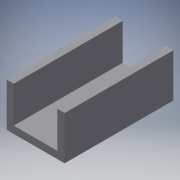
# Autodesk Inventor part: anclaje
Saved by Autodesk Inventor 2018 (Build 220112000, 112)
## iProperties
Created: 2021-07-06
Part Number: anclaje
Material: Genérico
Document SubType Name: Modeling
Designer: GABRIEL
Density: 1 g/cm^3
Appearance: Valor por defecto
Author: GABRIEL
Autodesk Inventor part; units mm, degrees
ref_plane "YZ Plane" through (0, 0, 0) normal (1, 0, 0) x (0, 1, 0)
ref_plane "XZ Plane" through (0, 0, 0) normal (0, 1, 0) x (-1, 0, 0)
ref_plane "XY Plane" through (0, 0, 0) normal (0, 0, 1) x (1, 0, 0)
sketch "Boceto1" plane through (0, 0, 0) normal (0, 1, 0) x (-1, 0, 0)
  line L0 (0, 0) -> (-80, 0)
  line L1 (-80, 0) -> (-80, -40)
  line L2 (-80, -40) -> (0, -40)
  line L3 (0, -40) -> (0, 0)
  line L4 (-10, 0) -> (-70, 0)
  line L5 (-70, 0) -> (-70, -30)
  line L6 (-70, -30) -> (-10, -30)
  line L7 (-10, -30) -> (-10, 0)
  dimension "d0" = 80
  dimension "d1" = 40
  dimension "d2" = 60
  dimension "d3" = 30
  constraints: 16 end point, 4 parallel, 2 horizontal, 2 perpendicular, 1 point on line
  measures "d0" distance of L2.end L1.end
  measures "d1" distance of L1.end L0.end
  measures "d2" distance of L6.end L5.end
  measures "d3" distance of L5.end L4.end
extrude "Extrusión1" add sketch "Boceto1" along normal blind 150 contours L3 L2 L1 L0 L5 L6 L7
sketch "Boceto2" plane through (80, 0, -40) normal (0, 0, -1) x (-1, 0, 0)
  circle A0 centre (40, 120) radius 10
  circle A1 centre (40, 30) radius 10
  line L0 (0, 0) -> (80, 0) projected
  line L1 (80, 0) -> (80, 150) projected
  circle A2 centre (40, 75) radius 12.5
  dimension "d6" = 20
  dimension "d7" = 20
  dimension "d8" = 120
  dimension "d9" = 40
  dimension "d10" = 40
  dimension "d11" = 25
  dimension "d12" = 40
  dimension "d13" = 75
  dimension "d14" = 30
  constraints: 3 centre point
  measures "d6" diameter of A0
  measures "d7" diameter of A1
  measures "d8" distance from line of L0 A0.centre
  measures "d9" distance from line of L1 A0.centre
  measures "d10" distance from line of L1 A1.centre
  measures "d11" diameter of A2
  measures "d12" distance from line of A2.centre L1
  measures "d13" distance from line of A2.centre L0
  measures "d14" distance from line of A1.centre L0
extrude "Extrusión2" cut sketch "Boceto2" against normal blind 150
